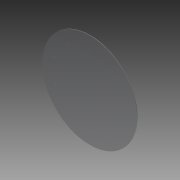
# Autodesk Inventor part: Plexiglas
Saved by Autodesk Inventor 2015 (Build 190159000, 159)
## iProperties
Created: 2018-03-07
Part Number: Plexiglas
Material: Plexiglas
Document SubType Name: Modeling
Designer: wepet
Density: 1.2 g/cm^3
Appearance: Polycarbonat - Rauch
Author: wepet
Autodesk Inventor part; units mm, degrees
ref_plane "YZ Plane" through (0, 0, 0) normal (1, 0, 0) x (0, 1, 0)
ref_plane "XZ Plane" through (0, 0, 0) normal (0, 1, 0) x (-1, 0, 0)
ref_plane "XY Plane" through (0, 0, 0) normal (0, 0, 1) x (1, 0, 0)
sketch "Skizze1" plane through (0, 0, 0) normal (0, 1, 0) x (-1, 0, 0)
  circle A0 centre (0, 0) radius 247.5
  dimension "d0" = 495
  constraints: 1 centre point, 1 coincident
  measures "d0" diameter of A0
extrude "Extrusion_grundplatte" add sketch "Skizze1" along normal blind 3
sketch "Skizze6" plane through (0, 0, 0) normal (0, -1, 0) x (1, 0, 0)
  circle A0 centre (0, 0) radius 247.5 projected
  line L0 (0, 0) -> (0, 190) construction
  line L1 (0, 0) -> (-111.6792, 153.7132) construction
  line L2 (0, 0) -> (-180.7007, 58.7132) construction
  line L3 (0, 0) -> (-180.7007, -58.7132) construction
  line L4 (0, 0) -> (-111.6792, -153.7132) construction
  line L5 (0, 0) -> (0, -190) construction
  line L6 (0, 0) -> (111.6792, -153.7132) construction
  line L7 (0, 0) -> (180.7007, -58.7132) construction
  line L8 (0, 0) -> (180.7007, 58.7132) construction
  line L9 (0, 0) -> (111.6792, 153.7132) construction
  dimension "d47" = 190
  dimension "d50" = 360
  constraints: 20 end point, 10 coincident, 1 vertical, 41 other
  measures "d47" distance of L0.start L0.end
hole "Bohrung_halter_plexiglas" at (0, 0, 190) at (-111.6792, 0, 153.7132) at (-180.7007, 0, 58.7132) at (-180.7007, 0, -58.7132) at (-111.6792, 0, -153.7132) at (0, 0, -190) at (111.6792, 0, -153.7132) at (180.7007, 0, -58.7132) at (180.7007, 0, 58.7132) at (111.6792, 0, 153.7132) direction (0, 1, 0) diameter 4 end through all
